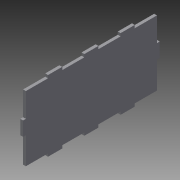
# Autodesk Inventor part: Стенка задняя
Saved by Autodesk Inventor 2022 (Build 260153000, 153)
## iProperties
RuleStatus: InUse
Part Number: Стенка задняя
Checked By: Якушев
Engr Approved By: Малов
Material: По умолчанию1
Document SubType Name: Modeling
Mfg Approved By: Судаков
Designer: Смирнов
Density: 1 g/cm^3
Appearance: По умолчанию1
AfterMaterialChange0: Материал
BeforeDocSave0: Материал
AfterAnyiPropertyChange0: Материал
Материал: По умолчанию1
Author: Смирнов
Autodesk Inventor part; units mm, degrees
ref_plane "YZ Plane" through (0, 0, 0) normal (1, 0, 0) x (0, 1, 0)
ref_plane "XY Plane" through (0, 0, 0) normal (0, 0, 1) x (1, 0, 0)
sketch "Эскиз1" plane through (0, 0, 0) normal (0, 0, 1) x (1, 0, 0)
  circle A0 centre (0, 0) radius 145
  line L0 (0, 145) -> (-243.8305, 145)
  line L1 (-243.8305, 145) -> (-243.8305, -145)
  line L2 (-243.8305, -145) -> (0, -145)
  line L3 (0, 0) -> (-278.593, 0) construction
  line L4 (0, 0) -> (0, 238.8567) construction
  circle A1 centre (-194.4152, 0) radius 49.4152 construction
  circle A2 centre (-169.2951, 95.5848) radius 49.4152 construction
  circle A3 centre (-169.2951, -95.5848) radius 49.4152 construction
  point P0 (145, 0)
  dimension "d4" = 290
  dimension "d5" = 388.8305
  constraints: 10 end point, 9 tangent, 4 centre point, 3 point on circle, 2 equal radius, 2 horizontal, 2 point on line, 1 coincident, 1 perpendicular, 1 vertical, 1 other
  measures "d4" diameter of A0
  measures "d5" distance from line of L1 point (145, 0)
extrude "Выдавливание1" add sketch "Эскиз1" along normal blind 6
sketch "Эскиз2" plane through (0, 0, 0) normal (0, 0, 1) x (1, 0, 0)
  line L0 (-243.8305, 145) -> (-243.8305, -145) construction
  line L1 (0, 145) -> (-243.8305, 145) construction
  line L2 (-243.8305, -145) -> (0, -145) construction
  line L3 (-243.8305, 145) -> (0, 145)
  line L4 (0, 145) -> (0, 139)
  line L5 (0, 139) -> (-243.8305, 139)
  line L6 (-243.8305, 139) -> (-243.8305, 145)
  line L7 (-243.8305, 145) -> (-237.8305, 145)
  line L8 (-237.8305, 145) -> (-237.8305, -145)
  line L9 (-237.8305, -145) -> (-243.8305, -145)
  line L10 (-243.8305, -145) -> (-243.8305, 145)
  point P0 (0, 0)
  dimension "d8" = 6
  dimension "d9" = 6
  constraints: 16 end point, 4 parallel, 2 horizontal, 2 perpendicular, 2 point on line
  measures "d8" distance between parallel lines of L1 L5
  measures "d9" distance between parallel lines of L0 L8
extrude "Выдавливание2" add sketch "Эскиз2" along normal blind 150 separate body contours L3 L8 L5 L6 | L3 L4 L5 L8
extrude "Выдавливание3" add sketch "Эскиз2" along normal blind 150 separate body contours L3 L8 L5 L6 | L5 L8 L9 L10
sketch "Эскиз3" plane through (0, 0, 0) normal (0, 0, 1) x (1, 0, 0)
  line L0 (0, 145) -> (0, 139) construction
  line L1 (0, 145) -> (-243.8305, 145) construction
  line L2 (0, 139) -> (-243.8305, 139) construction
  line L3 (-237.8305, 145) -> (-237.8305, -145) construction
  line L4 (-243.8305, 145) -> (-243.8305, -145) construction
  line L5 (-243.8305, -145) -> (0, -145) construction
  line L6 (0, 145) -> (-30, 145)
  line L7 (-30, 145) -> (-30, 139)
  line L8 (-30, 139) -> (0, 139)
  line L9 (0, 139) -> (0, 145)
  line L10 (-79, 145) -> (-109, 145)
  line L11 (-109, 145) -> (-109, 139)
  line L12 (-109, 139) -> (-79, 139)
  line L13 (-79, 139) -> (-79, 145)
  line L14 (-158, 145) -> (-188, 145)
  line L15 (-188, 145) -> (-188, 139)
  line L16 (-188, 139) -> (-158, 139)
  line L17 (-158, 139) -> (-158, 145)
  line L18 (-237.8305, 92) -> (-243.8305, 92)
  line L19 (-243.8305, 92) -> (-243.8305, 62)
  line L20 (-243.8305, 62) -> (-237.8305, 62)
  line L21 (-237.8305, 62) -> (-237.8305, 92)
  line L22 (0, 0) -> (-283.1064, 0) construction
  line L23 (-237.8305, 15) -> (-243.8305, 15)
  line L24 (-243.8305, 15) -> (-243.8305, -15)
  line L25 (-243.8305, -15) -> (-237.8305, -15)
  line L26 (-237.8305, -15) -> (-237.8305, 15)
  line L27 (-237.8305, -92) -> (-243.8305, -92)
  line L28 (-243.8305, -92) -> (-243.8305, -62)
  line L29 (-243.8305, -62) -> (-237.8305, -62)
  line L30 (-237.8305, -62) -> (-237.8305, -92)
  line L31 (0, -145) -> (0, -139) construction
  line L32 (0, -145) -> (-30, -145)
  line L33 (-30, -145) -> (-30, -139)
  line L34 (-30, -139) -> (0, -139)
  line L35 (0, -139) -> (0, -145)
  line L36 (-79, -145) -> (-109, -145)
  line L37 (-109, -145) -> (-109, -139)
  line L38 (-109, -139) -> (-79, -139)
  line L39 (-79, -139) -> (-79, -145)
  line L40 (-158, -145) -> (-188, -145)
  line L41 (-188, -145) -> (-188, -139)
  line L42 (-188, -139) -> (-158, -139)
  line L43 (-158, -139) -> (-158, -145)
  dimension "d14" = 49
  dimension "d15" = 49
  dimension "d16" = 30
  dimension "d17" = 47
  dimension "d19" = 47
  dimension "d20" = 49.8305
  constraints: 76 end point, 16 symmetric about line, 10 parallel, 9 point on line, 6 horizontal, 5 perpendicular, 4 equal length, 1 other
  measures "d14" distance between parallel lines of L13 L7
  measures "d15" distance between parallel lines of L17 L11
  measures "d16" distance between parallel lines of L0 L7
  measures "d17" distance between parallel lines of L18 L2
  measures "d19" distance from line of L23.start L20
  measures "d20" distance between parallel lines of L3 L15
extrude "Выдавливание4" cut sketch "Эскиз3" along normal through all bodies 1
sketch "Эскиз4" plane through (-243.8305, 145, 0) normal (0, 1, 0) x (1, 0, 0)
  line L0 (55.8305, -6) -> (55.8305, 0) projected
  line L1 (55.8305, 0) -> (0, 0) projected
  line L2 (0, 0) -> (0, -6) projected
  line L3 (55.8305, -6) -> (0, -6) projected
  line L4 (85.8305, 0) -> (85.8305, -6) projected
  line L5 (134.8305, -6) -> (85.8305, -6) projected
  line L6 (134.8305, -6) -> (134.8305, 0) projected
  line L7 (134.8305, 0) -> (85.8305, 0) projected
  line L8 (164.8305, 0) -> (164.8305, -6) projected
  line L9 (213.8305, -6) -> (164.8305, -6) projected
  line L10 (213.8305, -6) -> (213.8305, 0) projected
  line L11 (213.8305, 0) -> (164.8305, 0) projected
  point P0 (243.8305, 0)
extrude "Выдавливание5" cut sketch "Эскиз4" against normal through all bodies 2
sketch "Эскиз5" plane through (-243.8305, -145, 0) normal (-1, 0, 0) x (0, 0, 1)
  line L0 (0, 237) -> (6, 237) projected
  line L1 (6, 290) -> (6, 237) projected
  line L2 (0, 290) -> (6, 290) projected
  line L3 (0, 290) -> (0, 237) projected
  line L4 (6, 207) -> (0, 207) projected
  line L5 (0, 207) -> (0, 160) projected
  line L6 (0, 160) -> (6, 160) projected
  line L7 (6, 207) -> (6, 160) projected
  line L8 (6, 130) -> (0, 130) projected
  line L9 (0, 130) -> (0, 83) projected
  line L10 (0, 83) -> (6, 83) projected
  line L11 (6, 130) -> (6, 83) projected
  line L12 (6, 53) -> (0, 53) projected
  line L13 (0, 53) -> (0, 0) projected
  line L14 (0, 0) -> (6, 0) projected
  line L15 (6, 53) -> (6, 0) projected
  point P0 (0, 145)
extrude "Выдавливание6" cut sketch "Эскиз5" against normal through all bodies 3
sketch "Эскиз6" plane through (-243.8305, 145, 150) normal (0, 1, 0) x (1, 0, 0)
  line L0 (0, 144) -> (0, 0) construction
  line L1 (0, 57) -> (6, 57)
  line L2 (6, 57) -> (6, 87)
  line L3 (6, 87) -> (0, 87)
  line L4 (0, 87) -> (0, 57)
  point P0 (243.8305, 150)
  point P1 (0, 72)
  dimension "d27" = 30
  dimension "d28" = 6
  constraints: 8 end point, 2 midpoint, 2 parallel, 1 horizontal, 1 perpendicular, 1 point on line
  measures "d27" distance of L1.end L2.end
  measures "d28" distance of L1.start L1.end
extrude "Выдавливание7" cut sketch "Эскиз6" against normal through all bodies 2
sketch "Эскиз7" plane through (-243.8305, -145, 150) normal (-1, 0, 0) x (0, 0, 1)
  line L0 (-57, 290) -> (-57, 284) projected
  line L1 (-57, 284) -> (0, 284) projected
  line L2 (0, 290) -> (0, 284) projected
  line L3 (-57, 290) -> (0, 290) projected
  line L4 (-87, 284) -> (-87, 290) projected
  line L5 (-144, 290) -> (-87, 290) projected
  line L6 (-144, 290) -> (-144, 284) projected
  line L7 (-144, 284) -> (-87, 284) projected
  point P0 (-150, 145)
extrude "Выдавливание8" cut sketch "Эскиз7" against normal through all bodies 3
mirror "Зеркальное отражение2" about plane through (0, 0, 0) normal (0, 1, 0) of "Выдавливание8" bodies 3
ref_plane "РабПлоскость1" through (0, 0, 75) normal (0, 0, 1) x (1, 0, 0)
mirror "Зеркальное отражение3" about plane through (0, 0, 75) normal (0, 0, 1) of "Выдавливание5" bodies 2
mirror "Зеркальное отражение4" about plane through (0, 0, 75) normal (0, 0, 1) of "Выдавливание6" bodies 3
mirror "Зеркальное отражение5" about plane through (0, 0, 0) normal (0, 1, 0) bodies 2 separate body
sketch "Эскиз8" plane through (-243.8305, 62, 144) normal (0, 0, 1) x (1, 0, 0)
  line L0 (55.8305, 83) -> (55.8305, 77) projected
  line L1 (55.8305, 77) -> (85.8305, 77) projected
  line L2 (85.8305, 77) -> (85.8305, 83) projected
  line L3 (134.8305, 83) -> (85.8305, 83) projected
  line L4 (134.8305, 83) -> (134.8305, 77) projected
  line L5 (134.8305, 77) -> (164.8305, 77) projected
  line L6 (164.8305, 77) -> (164.8305, 83) projected
  line L7 (213.8305, 83) -> (164.8305, 83) projected
  line L8 (213.8305, 83) -> (213.8305, 77) projected
  line L9 (213.8305, 77) -> (243.8305, 77) projected
  line L10 (243.8305, 77) -> (243.8305, 83) projected
  arc A0 (243.8305, -207) -> (243.8305, 83) centre (243.8305, -62) ccw projected
  line L11 (243.8305, -207) -> (243.8305, -201) projected
  line L12 (243.8305, -201) -> (213.8305, -201) projected
  line L13 (213.8305, -201) -> (213.8305, -207) projected
  line L14 (164.8305, -207) -> (213.8305, -207) projected
  line L15 (164.8305, -207) -> (164.8305, -201) projected
  line L16 (164.8305, -201) -> (134.8305, -201) projected
  line L17 (134.8305, -201) -> (134.8305, -207) projected
  line L18 (85.8305, -207) -> (134.8305, -207) projected
  line L19 (85.8305, -207) -> (85.8305, -201) projected
  line L20 (85.8305, -201) -> (55.8305, -201) projected
  line L21 (55.8305, -201) -> (55.8305, -207) projected
  line L22 (0, -207) -> (55.8305, -207) projected
  line L23 (0, -154) -> (0, -207) projected
  line L24 (0, -154) -> (6, -154) projected
  line L25 (6, -154) -> (6, -124) projected
  line L26 (6, -124) -> (0, -124) projected
  line L27 (0, -77) -> (0, -124) projected
  line L28 (0, -77) -> (6, -77) projected
  line L29 (6, -77) -> (6, -47) projected
  line L30 (6, -47) -> (0, -47) projected
  line L31 (0, 0) -> (0, -47) projected
  line L32 (0, 0) -> (6, 0) projected
  line L33 (6, 0) -> (6, 30) projected
  line L34 (6, 30) -> (0, 30) projected
  line L35 (0, 83) -> (0, 30) projected
  line L36 (55.8305, 83) -> (0, 83) projected
extrude "Выдавливание9" add sketch "Эскиз8" along normal blind 6 separate body
sketch "Эскиз9" plane through (0, 0, 6) normal (0, 0, 1) x (1, 0, 0)
  arc A0 (0, -145) -> (0, 145) centre (0, 0) ccw projected
  line L0 (0, -145) -> (0, -139) projected
  line L1 (0, 139) -> (0, 145) projected
  circle A1 centre (0, 0) radius 139
  constraints: 1 coincident, 3 other
extrude "Выдавливание10" add sketch "Эскиз9" along normal up to surface (138 mm away) separate body contours L0 A1 L1 A0
sketch "Эскиз12" plane through (-243.8305, 62, 150) normal (0, 0, 1) x (1, 0, 0)
  line L0 (243.8305, -62) -> (418.5063, -62) construction
  line L1 (243.8305, -62) -> (367.9586, 42.1558)
  line L2 (243.8305, -62) -> (323.5999, 76.1647)
  arc A0 (243.8305, -207) -> (243.8305, 83) centre (243.8305, -62) ccw projected
  arc A1 (243.8305, -201) -> (243.8305, 77) centre (243.8305, -62) ccw projected
  point P0 (313.3305, 58.3775)
  point P1 (350.3107, 27.3475)
  point P2 (354.9069, 31.2042)
  point P3 (316.3305, 63.5737)
  dimension "d44" = 20
  dimension "d45" = 40
  constraints: 6 end point, 1 horizontal
  measures "d44" angle of L1 L2
  measures "d45" angle of L0 L1
extrude "Выдавливание13" cut sketch "Эскиз12" against normal through all contours A1 L2 A0 L1 bodies 5
mirror "Зеркальное отражение7" about plane through (0, 0, 0) normal (0, 1, 0) of "Выдавливание13" bodies 5
sketch "Эскиз13" plane through (0, 0, 144) normal (0, 0, 1) x (1, 0, 0)
  arc A0 (0, -145) -> (0, 145) centre (0, 0) ccw projected
  line L0 (0, 139) -> (0, 145) projected
  arc A1 (0, -139) -> (0, 139) centre (0, 0) ccw projected
  line L1 (0, -145) -> (0, -139) projected
  line L2 (111.0764, 93.2042) -> (106.4802, 89.3475) projected
  line L3 (69.5, 120.3775) -> (72.5, 125.5737) projected
  line L4 (72.5, -125.5737) -> (69.5, -120.3775) projected
  line L5 (106.4802, -89.3475) -> (111.0764, -93.2042) projected
extrude "Выдавливание14" add sketch "Эскиз13" along normal blind 6 contours L4 A1 L5 A0 | L2 A1 L3 A0 bodies 6
sketch "Эскиз10" plane through (0, 0, 144) normal (0, 0, 1) x (1, 0, 0)
  line L0 (-175.9322, -50) -> (175.9322, -50)
  line L1 (175.9322, -50) -> (175.9322, 50)
  line L2 (175.9322, 50) -> (-175.9322, 50)
  line L3 (-175.9322, 50) -> (-175.9322, -50)
  line L4 (-175.9322, -50) -> (175.9322, 50) construction
  line L5 (175.9322, -50) -> (-175.9322, 50) construction
  point P0 (0, 0)
  dimension "d37" = 100
  constraints: 12 end point, 2 midpoint, 2 parallel, 1 horizontal, 1 perpendicular
  measures "d37" distance of L0.end L1.end
extrude "Выдавливание11" cut sketch "Эскиз10" against normal through all bodies 6
sketch "Эскиз11" plane through (-243.8305, 62, 150) normal (0, 0, 1) x (1, 0, 0)
  line L0 (373.5263, -112) -> (379.9371, -112) projected
  line L1 (379.9371, -12) -> (373.5263, -12) projected
  circle A0 centre (338.8305, -62) radius 50
  line L2 (379.9371, -12) -> (338.8305, -12)
  line L3 (379.9371, -112) -> (338.8305, -112)
  circle A1 centre (338.8305, -62) radius 26.5 construction
  arc A2 (243.8305, -207) -> (243.8305, 83) centre (243.8305, -62) ccw projected
  dimension "d40" = 53
  constraints: 4 end point, 4 tangent, 2 centre point, 2 point on circle, 1 coincident, 1 collinear
  measures "d40" diameter of A1
extrude "Выдавливание12" cut sketch "Эскиз11" against normal through all bodies 5
sketch "Эскиз14" plane through (0, 0, 6) normal (0, 0, -1) x (-1, 0, 0)
  line L0 (0, 0) -> (-32.4582, 184.0794) construction
  line L1 (0, 0) -> (-150.2309, 86.7358) construction
  line L2 (0, 0) -> (-110.9269, 158.42) construction
  line L3 (0, 0) -> (-198.0131, 0) construction
  arc A0 (0, 139) -> (-129.6958, 50) centre (0, 0) ccw construction
  circle A1 centre (-24.1371, 136.8883) radius 6
  circle A2 centre (-79.7271, 113.8621) radius 6
  circle A3 centre (-120.3775, 69.5) radius 6
  arc A4 (-136.1066, -50) -> (0, -145) centre (0, 0) ccw construction
  point P0 (-135.0734, 52.7273)
  point P1 (0, 145)
  dimension "d50" = 25
  dimension "d51" = 55
  dimension "d52" = 12
  constraints: 8 end point, 3 centre point, 3 point on circle, 3 point on line, 2 equal radius, 1 horizontal, 1 tangent, 1 other
  measures "d50" angle of L0 L2
  measures "d51" angle of L3 L2
  measures "d52" diameter of A1
extrude "Выдавливание15" add sketch "Эскиз14" against normal blind 10 bodies 6
fillet "Сопряжение2" radius 5 6 edges at (18.2071, 137.8024, 11) (30.0221, 135.7191, 11) (74.7391, 117.1967, 11) (84.5666, 110.3154, 11) (117.2661, 74.6302, 11) (123.2647, 64.2403, 11)
sketch "Эскиз15" plane through (0, 0, 6) normal (0, 0, -1) x (-1, 0, 0)
  arc A0 (-28.7951, 133.1063) -> (-18.4665, 134.9275) centre (-24.1371, 136.8883) ccw projected
  arc A1 (-82.3504, 108.466) -> (-73.7592, 114.4816) centre (-79.7271, 113.8621) ccw projected
  arc A2 (-120.4745, 63.5008) -> (-115.2305, 72.5836) centre (-120.3775, 69.5) ccw projected
  point P0 (0, 0)
hole "Отверстие1" at (24.1371, 136.8883, 6) at (79.7271, 113.8621, 6) at (120.3775, 69.5, 6) direction (0, 0, 1) diameter 3.9 depth 9 countersink diameter 4.5 countersink angle 90 bodies 6
mirror "Зеркальное отражение9" about plane through (0, 0, 0) normal (0, 1, 0) of "Отверстие1", "Выдавливание15", "Сопряжение2" bodies 6
sketch "Эскиз16" plane through (0, 0, 0) normal (0, 0, -1) x (-1, 0, 0)
  circle A0 centre (-24.1371, -136.8883) radius 1.95 construction
  circle A1 centre (-79.7271, -113.8621) radius 1.95 construction
  circle A2 centre (-79.7271, -113.8621) radius 1.95 construction
  circle A3 centre (-120.3775, -69.5) radius 1.95 construction
  circle A4 centre (-120.3775, -69.5) radius 1.95 construction
  circle A5 centre (-120.3775, 69.5) radius 1.95 construction
  circle A6 centre (-120.3775, 69.5) radius 1.95 construction
  circle A7 centre (-79.7271, 113.8621) radius 1.95 construction
  circle A8 centre (-79.7271, 113.8621) radius 1.95 construction
  circle A9 centre (-24.1371, 136.8883) radius 1.95 construction
  circle A10 centre (-24.1371, 136.8883) radius 1.95 construction
  circle A11 centre (-120.3775, -69.5) radius 1.6
  circle A12 centre (-79.7271, -113.8621) radius 1.6
  circle A13 centre (-24.1371, -136.8883) radius 1.6
  circle A14 centre (-120.3775, 69.5) radius 1.6
  circle A15 centre (-79.7271, 113.8621) radius 1.6
  circle A16 centre (-24.1371, 136.8883) radius 1.6
  point P0 (0, 0)
  dimension "d63" = 3.2
  constraints: 6 centre point, 6 coincident, 5 equal radius
  measures "d63" diameter of A16
extrude "Выдавливание16" cut sketch "Эскиз16" against normal through all bodies 1
ref_plane "РабПлоскость2" through (5.15, 0, 128) normal (0, 0, 1) x (-1, 0, 0)
sketch "Эскиз17" plane through (5.15, 0, 128) normal (0, 0, 1) x (-1, 0, 0)
  arc A0 (-11.25, -5.1) -> (-10.25, -6.1) centre (-10.25, -5.1) ccw projected
  line L0 (-10.25, -6.1) -> (10.25, -6.1) projected
  arc A1 (10.25, -6.1) -> (11.25, -5.1) centre (10.25, -5.1) ccw projected
  line L1 (11.25, -5.1) -> (11.25, 5.1) projected
  arc A2 (11.25, 5.1) -> (10.25, 6.1) centre (10.25, 5.1) ccw projected
  line L2 (10.25, 6.1) -> (-10.25, 6.1) projected
  arc A3 (-10.25, 6.1) -> (-11.25, 5.1) centre (-10.25, 5.1) ccw projected
  line L3 (-11.25, 5.1) -> (-11.25, -5.1) projected
  line L4 (31.25, -12.1) -> (-17.25, -12.1)
  line L5 (-17.25, -12.1) -> (-17.25, 12.1)
  line L6 (-17.25, 12.1) -> (31.25, 12.1)
  line L7 (31.25, 12.1) -> (31.25, -12.1)
  line L8 (5.15, 0) -> (-37.4829, 0) construction
  line L9 (31.25, -12.1) -> (31.25, -139)
  line L10 (31.25, -139) -> (7, -139)
  line L11 (7, -139) -> (7, -12.1)
  line L12 (35.15, -139) -> (5.15, -139) construction
  line L13 (31.25, 12.1) -> (31.25, 139)
  line L14 (31.25, 139) -> (7, 139)
  line L15 (7, 139) -> (7, 12.1)
  line L16 (35.15, 139) -> (5.15, 139) construction
  arc A4 (14.766, 0.5) -> (14.766, -0.5) centre (13.9, 0) ccw projected
  arc A5 (-14.766, -0.5) -> (-14.766, 0.5) centre (-13.9, 0) ccw projected
  circle A6 centre (13.9, 0) radius 0.95
  circle A7 centre (-13.9, 0) radius 0.95
  line L17 (11.25, 2.5) -> (12.25, 2.5)
  line L18 (12.25, 2.5) -> (12.25, -2.5)
  line L19 (12.25, -2.5) -> (11.25, -2.5)
  line L20 (11.25, -2.5) -> (11.25, 2.5)
  point P0 (7, 12.1)
  dimension "d66" = 6
  dimension "d67" = 6
  dimension "d68" = 20
  dimension "d69" = 1.9
  dimension "d73" = 5
  dimension "d74" = 1
  constraints: 32 end point, 5 symmetric about line, 4 parallel, 4 perpendicular, 3 horizontal, 2 centre point, 2 coincident, 2 midpoint, 1 collinear, 1 equal radius, 1 point on line, 1 vertical, 2 other
  measures "d66" distance between parallel lines of L5 L3
  measures "d67" distance between parallel lines of L4 L0
  measures "d68" distance between parallel lines of L1 L7
  measures "d69" diameter of A6
  measures "d73" distance of L17.end L18.end
  measures "d74" distance of L17.start L17.end
extrude "Выдавливание17" add sketch "Эскиз17" along normal blind 6 separate body
fillet "Сопряжение3" radius 5 2 edges at (22.4, -12.1, 131) (22.4, 12.1, 131)
fillet "Сопряжение3" radius 10 2 edges at (-1.85, 12.1, 131) (-1.85, -12.1, 131)
sketch "Эскиз18" plane through (0, 145, 150) normal (0, 1, 0) x (1, 0, 0)
  line L0 (-27.975, 24) -> (-25.975, 22) construction
  line L1 (-27.975, 27) -> (-27.975, 24) construction
  arc A0 (-24.975, 30) -> (-27.975, 27) centre (-24.975, 27) ccw construction
  line L2 (-2.975, 30) -> (-24.975, 30) construction
  arc A1 (0.025, 27) -> (-2.975, 30) centre (-2.975, 27) ccw construction
  line L3 (0.025, 11) -> (0.025, 27) construction
  arc A2 (-2.975, 8) -> (0.025, 11) centre (-2.975, 11) ccw construction
  line L4 (-24.975, 8) -> (-2.975, 8) construction
  arc A3 (-27.975, 11) -> (-24.975, 8) centre (-24.975, 11) ccw construction
  line L5 (-27.975, 14) -> (-27.975, 11) construction
  line L6 (-25.975, 16) -> (-27.975, 14) construction
  line L7 (-1.85, 16) -> (-25.975, 16) construction
  line L8 (-1.85, 22) -> (-1.85, 16) construction
  line L9 (-25.975, 22) -> (-1.85, 22) construction
  circle A4 centre (-22.975, 26) radius 1.95 construction
  circle A5 centre (-4.975, 26) radius 1.95 construction
  circle A6 centre (-4.975, 12) radius 1.95 construction
  circle A7 centre (-22.975, 12) radius 1.95 construction
  circle A8 centre (-4.975, 12) radius 1.6
  circle A9 centre (-22.975, 12) radius 1.6
  circle A10 centre (-22.975, 26) radius 1.6
  circle A11 centre (-4.975, 26) radius 1.6
  point P0 (0, 150)
  dimension "d76" = 3.2
  constraints: 4 centre point, 4 coincident, 3 equal radius
  measures "d76" diameter of A10
extrude "Выдавливание18" cut sketch "Эскиз18" against normal through all bodies 2 4
sketch "Эскиз19" plane through (-243.8305, 62, 150) normal (0, 0, 1) x (1, 0, 0)
  line L0 (243.8305, -62) -> (-34.9022, -62) construction
  circle A0 centre (74.5354, -157.5848) radius 49.4152 construction
  circle A1 centre (49.4152, -62) radius 49.4152 construction
  circle A2 centre (74.5354, 33.5848) radius 49.4152 construction
  circle A3 centre (74.5354, 33.5848) radius 35
  circle A4 centre (49.4152, -62) radius 35
  circle A5 centre (74.5354, -157.5848) radius 35
  dimension "d79" = 70
  constraints: 3 centre point, 3 coincident, 2 end point, 2 equal radius, 1 horizontal
  measures "d79" diameter of A3
extrude "Выдавливание19" cut sketch "Эскиз19" against normal through all bodies 5
sketch "Эскиз20" plane through (0, 0, 0) normal (0, 0, -1) x (-1, 0, 0)
  circle A0 centre (0, 0) radius 90 construction
  line L0 (0, 0) -> (-250.4545, 0) construction
  point P0 (-90, 0)
  point P1 (0, -90)
  point P2 (90, 0)
  point P3 (0, 90)
  dimension "d82" = 180
  dimension "d85" = 360
  constraints: 2 end point, 1 coincident, 1 horizontal, 1 horizontal alignment, 1 point on line, 7 other
hole "Отверстие2" at (90, 0, 0) at (0, -90, 0) at (-90, 0, 0) at (0, 90, 0) direction (0, 0, 1) diameter 3.4 end through all bodies 1
sketch "Эскиз21" plane through (0, 0, 0) normal (0, 0, -1) x (-1, 0, 0)
  circle A0 centre (0.25, 15) radius 1.7 projected
  circle A1 centre (-19.75, 15) radius 1.7 projected
  circle A2 centre (-19.75, -15) radius 1.7 projected
  circle A3 centre (0.25, -15) radius 1.7 projected
  point P0 (0, 0)
extrude "Выдавливание20" cut sketch "Эскиз21" against normal through all bodies 1
sketch "Эскиз22" plane through (0, 0, 6) normal (0, 0, 1) x (1, 0, 0)
  arc A0 (0, -145) -> (0, 145) centre (0, 0) ccw projected
  arc A1 (106.4802, -89.3475) -> (129.6958, -50) centre (0, 0) ccw projected
  circle A2 centre (0, 0) radius 139
  line L0 (136.1066, -50) -> (95, -50) projected
  line L1 (95, 50) -> (136.1066, 50) projected
  point P0 (129.6958, 50)
  constraints: 1 coincident, 3 other
extrude "Выдавливание21" add sketch "Эскиз22" along normal blind 75 separate body contours L0 A2 L1 A0
sketch "Эскиз23" plane through (0, 0, 6) normal (0, 0, -1) x (-1, 0, 0)
  circle A0 centre (-139, 0) radius 6
  arc A1 (-136.1066, 50) -> (-136.1066, -50) centre (0, 0) ccw construction
  line L0 (0, 0) -> (-163.7686, 0) construction
  dimension "d98" = 12
  constraints: 2 end point, 1 centre point, 1 horizontal, 1 point on line, 1 tangent
  measures "d98" diameter of A0
extrude "Выдавливание22" add sketch "Эскиз23" against normal up to surface (10 mm away) bodies 8
fillet "Сопряжение4" radius 5 2 edges at (138.8705, -5.9986, 11) (138.8705, 5.9986, 11)
sketch "Эскиз24" plane through (0, 0, 6) normal (0, 0, -1) x (-1, 0, 0)
  arc A0 (-136.0844, -5.244) -> (-136.0844, 5.244) centre (-139, 0) ccw construction
  point P0 (0, 0)
hole "Отверстие3" at (139, 0, 6) direction (0, 0, 1) diameter 3.9 depth 8 countersink diameter 4.5 countersink angle 90 bodies 8
sketch "Эскиз25" plane through (0, 0, 0) normal (0, 0, -1) x (-1, 0, 0)
  circle A0 centre (-139, 0) radius 2.25 construction
  circle A1 centre (-139, 0) radius 1.7
  point P0 (0, 0)
  dimension "d109" = 3.4
  constraints: 1 centre point, 1 coincident
  measures "d109" diameter of A1
extrude "Выдавливание23" cut sketch "Эскиз25" against normal through all bodies 1
sketch "Эскиз26" plane through (-243.8305, 62, 144) normal (0, 0, -1) x (-1, 0, 0)
  line L0 (-379.9371, -112) -> (-338.8305, -112) projected
  arc A0 (-338.8305, -112) -> (-338.8305, -12) centre (-338.8305, -62) ccw projected
  line L1 (-338.8305, -12) -> (-379.9371, -12) projected
  line L2 (-379.9371, -6) -> (-338.8305, -6)
  arc A1 (-338.8305, -118) -> (-338.8305, -6) centre (-338.8305, -62) ccw
  line L3 (-338.8305, -118) -> (-379.9371, -118)
  circle A2 centre (-243.8305, -62) radius 138.5
  point P0 (-372.9903, -112)
  point P1 (-370.5043, -118)
  point P2 (-370.5043, -6)
  point P3 (-372.9903, -12)
  dimension "d112" = 6
  dimension "d113" = 277
  constraints: 4 end point, 2 centre point, 2 point on circle, 1 coincident, 2 other
  measures "d112" distance between parallel lines of L1 L2
  measures "d113" diameter of A2
extrude "Выдавливание24" add sketch "Эскиз26" along normal up to surface (63 mm away) separate body contours L0 A0 L1 A2 L2 A1 L3
sketch "Эскиз28" plane through (-243.8305, 62, 144) normal (0, 0, 1) x (1, 0, 0)
  line L0 (370.5043, -118) -> (338.8305, -118) projected
  line L1 (338.8305, -6) -> (370.5043, -6) projected
  arc A0 (379.9371, -112) -> (379.9371, -12) centre (243.8305, -62) ccw projected
  circle A1 centre (243.8305, -62) radius 138.5
  arc A2 (338.8305, -6) -> (338.8305, -118) centre (338.8305, -62) ccw projected
  line L2 (356.4101, 18.6727) -> (306.7102, -16.1275)
  line L3 (338.8305, -62) -> (449.1874, -62) construction
  line L4 (356.4101, -142.6727) -> (306.7102, -107.8725)
  dimension "d121" = 35
  constraints: 6 end point, 3 point on circle, 2 symmetric about line, 1 centre point, 1 coincident, 1 horizontal, 1 tangent
  measures "d121" angle of L3 L2
extrude "Выдавливание25" add sketch "Эскиз28" against normal up to surface (63 mm away) contours A1 L4 A2 L0 | A1 L1 A2 L2 bodies 9
sketch "Эскиз27" plane through (0, 0, 0) normal (0, 1, 0) x (-1, 0, 0)
  line L0 (-74, 81) -> (-128, 81)
  line L1 (-128, 81) -> (-128, 111)
  line L2 (-128, 111) -> (-74, 111)
  line L3 (-74, 111) -> (-74, 81)
  line L4 (-45, 81) -> (-95, 81) construction
  line L5 (-101, 111) -> (-101, 42.3727) construction
  line L6 (0, 0) -> (0, 175.156)
  dimension "d116" = 202
  dimension "d117" = 54
  dimension "d118" = 30
  constraints: 12 end point, 2 parallel, 2 vertical, 1 collinear, 1 horizontal, 1 midpoint, 1 perpendicular
  measures "d116" diameter of L5 L6
  measures "d117" distance of L1.end L2.end
  measures "d118" distance of L0.end L1.end
revolve "Вращение1" cut sketch "Эскиз27" angle 360 about axis through (0, 0, 0) along (0, 0, 1) bodies 9
fillet "Сопряжение5" radius 5 4 edges at (61.5405, -41.0946, 81) (61.5405, 41.0946, 81) (111.5869, -62.7086, 81) (111.5869, 62.7086, 81)
ref_plane "РабПлоскость3" through (0, 0, 0) normal (-0.5, -0.8660254, 0) x (0, 0, 1)
sketch "Эскиз29" plane through (0, 0, 0) normal (-0.5, -0.8660254, 0) x (0, 0, 1)
  line L0 (136, -164.7493) -> (136, -126.8636) construction
  line L1 (137.95, -138.5) -> (137.95, -128.5)
  line L2 (137.95, -128.5) -> (136, -128.5)
  line L3 (137.95, -138.5) -> (136, -138.5)
  line L4 (136, -138.5) -> (136, -128.5)
  line L5 (144, -138.5) -> (81, -138.5) construction
  line L6 (144, -77.3917) -> (144, -137.8331) projected
  line L7 (137.7, -142.5) -> (137.7, -138.5)
  line L8 (137.95, -138.5) -> (137.7, -138.5)
  line L9 (6, -145) -> (144, -145) construction
  line L10 (137.7, -142.5) -> (140.2, -145)
  line L11 (140.2, -145) -> (136, -145)
  line L12 (136, -145) -> (136, -138.5)
  point P0 (0, 0)
  dimension "d125" = 3.9
  dimension "d126" = 8
  dimension "d127" = 10
  dimension "d128" = 3.4
  dimension "d129" = 135
  dimension "d130" = 2.5
  constraints: 20 end point, 6 point on line, 4 perpendicular, 2 collinear, 2 vertical, 1 horizontal
  measures "d125" diameter of L1 L0
  measures "d126" distance between parallel lines of L6 L0
  measures "d127" distance of L1.start L1.end
  measures "d128" diameter of L7 L0
  measures "d129" angle of L7 L10
  measures "d130" distance from line of L7.start L9
revolve "Вращение2" cut sketch "Эскиз29" angle 360 about axis through (142.6771, -82.3747, 136) along (-0.8660254, 0.5, 0) bodies 9 6
pattern_linear "Прямоуг.массив1" count 2 spacing 20 along (0, 0, -1) of "Вращение2" bodies 6 9
mirror "Зеркальное отражение10" about plane through (0, 0, 0) normal (0, 1, 0) of "Вращение2", "Прямоуг.массив1" bodies 6 9
sketch "Эскиз30" plane through (0, 0, 0) normal (0, 0, -1) x (-1, 0, 0)
  circle A0 centre (175.3305, -25) radius 1.7 construction
  circle A1 centre (175.3305, 25) radius 1.7 construction
  circle A2 centre (225.3305, 25) radius 1.7 construction
  circle A3 centre (225.3305, -25) radius 1.7 construction
  point P0 (0, 0)
hole "Отверстие4" at (-175.3305, 25, 0) at (-225.3305, 25, 0) at (-225.3305, -25, 0) at (-175.3305, -25, 0) direction (0, 0, 1) diameter 3.4 end through all bodies 1 clearance for "болты с шестигранной головкой / гайка ГОСТ 12876-67" size "M3" standard "ГОСТ"
pattern_circular "Круговой массив1" count 3 over 56 about axis through (0, 0, -10) along (0, 0, 1) of "Отверстие4" both ways yes bodies 1
split body "Разделение1" result two bodies by plane through (0, 0, 0) normal (0, 1, 0) bodies 6 first body at (93.6853, 110.015, 102)
equation "\"d15\" = d14"
